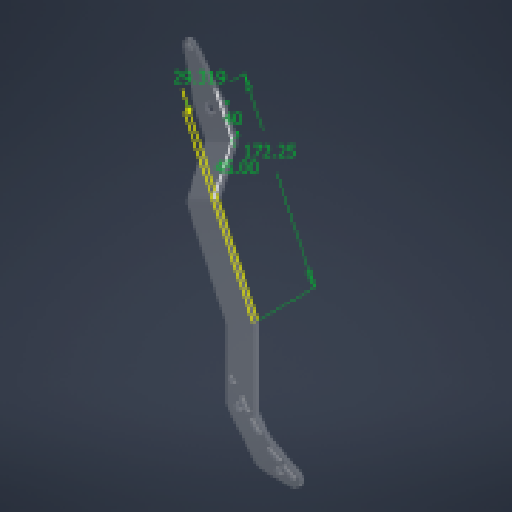
# Autodesk Inventor part: INTAKE_DROPPER_PLATE_SIDE
Saved by Autodesk Inventor 2026.2 (Build 302298010, 298A)
## iProperties
Created: 2026-04-03
Part Number: INTAKE_DROPPER_PLATE_SIDE
Material: Polycarbonate, Clear
Document SubType Name: Sheet Metal
Designer: 4aida
Density: 1.2 g/cm^3
Sheet Metal Rule: Default_mm
Appearance: Polycarbonate - Clear
Author: 4aida
Autodesk Inventor part; units mm, degrees
ref_plane "YZ Plane" through (0, 0, 0) normal (1, 0, 0) x (0, 1, 0)
ref_plane "XZ Plane" through (0, 0, 0) normal (0, 1, 0) x (-1, 0, 0)
ref_plane "XY Plane" through (0, 0, 0) normal (0, 0, 1) x (1, 0, 0)
sketch "Sketch6" plane through (5.547, -11.9185, -29.5428) normal (-0.0007043, -0.0003281, 0.9999997) x (0.9064037, 0.4224119, 0.0007769)
  circle A0 centre (0, 50) radius 3
  circle A1 centre (0, 50) radius 6
  line L0 (5.8818, 51.185) -> (16.194, 0)
  line L1 (16.194, 0) -> (-16.194, 0)
  line L2 (-16.194, 0) -> (-5.8818, 51.185)
  arc A2 (15.875, 0.0087) -> (-15.875, 0.0087) centre (0, 0) ccw
  point P0 (0.0297, 13.1461)
  point P1 (-15.5623, 3.1353)
  point P2 (15.5623, 3.1353)
  dimension "d68" = 6
  dimension "d69" = 12
  dimension "d70" = 50
  measures "d68" diameter of A0
  measures "d69" diameter of A1
  measures "d70" distance of A2.centre A0.centre
sketch "Sketch1" plane through (0, 0, 0) normal (0, 0, 1) x (1, 0, 0)
  circle A0 centre (0, 0) radius 2.4384
  circle A1 centre (0, 0) radius 15.875
  line L0 (-14.395, -6.6933) -> (56.9691, -160.1742)
  line L1 (90.6025, -274.8968) -> (130.7528, -274.8968)
  line L2 (86.9691, -148.9425) -> (14.3876, 6.7091)
  line L3 (129.6597, -266.3023) -> (96.0194, -248.4154)
  line L4 (96.0194, -248.4154) -> (72.0423, -218.8061)
  line L5 (72.0423, -218.8061) -> (69.5749, -220.8042) construction
  line L6 (69.5749, -220.8042) -> (93.9585, -250.9155)
  line L7 (93.9585, -250.9155) -> (128.1691, -269.1056)
  line L8 (128.1691, -269.1056) -> (129.6597, -266.3023) construction
  line L9 (74.4494, -236.9141) -> (67.2074, -238.0611)
  line L10 (67.2074, -238.0611) -> (62.593, -232.3628)
  line L11 (62.593, -232.3628) -> (65.2206, -225.5175)
  line L12 (65.2206, -225.5175) -> (72.4627, -224.3704)
  line L13 (72.4627, -224.3704) -> (77.0771, -230.0687) construction
  line L14 (77.0771, -230.0687) -> (74.4494, -236.9141)
  line L15 (112.0091, -274.8968) -> (105.535, -271.4545)
  line L16 (105.535, -271.4545) -> (105.2791, -264.1266)
  line L17 (105.2791, -264.1266) -> (111.4973, -260.2411)
  line L18 (111.4973, -260.2411) -> (117.9714, -263.6834) construction
  line L19 (117.9714, -263.6834) -> (118.2273, -271.0113)
  line L20 (118.2273, -271.0113) -> (112.0091, -274.8968)
  line L21 (128.1691, -269.1056) -> (106.6818, -269.1056) construction
  line L22 (5.0853, -149.4208) -> (51.9691, -149.4208) construction
  line L23 (51.9691, -149.4208) -> (51.9691, -259.6568) construction
  line L24 (51.9691, -259.6568) -> (5.0853, -259.6568) construction
  line L25 (5.0853, -259.6568) -> (5.0853, -149.4208) construction
  line L26 (-7.7017, -21.0883) -> (-3.3832, -19.0803)
  line L27 (-1.2744, -19.8505) -> (-1.2744, -19.8505)
  line L28 (-2.0446, -21.9593) -> (-6.3631, -23.9673)
  arc A2 (-1.2744, -19.8505) -> (-3.3832, -19.0803) centre (-2.7139, -20.5198) ccw
  arc A3 (-2.0446, -21.9593) -> (-1.2744, -19.8505) centre (-2.7139, -20.5198) ccw
  line L29 (130.7528, -274.8968) -> (136.4218, -264.2349)
  line L30 (136.4218, -264.2349) -> (99.265, -244.4782)
  line L31 (99.265, -244.4782) -> (86.9691, -229.2942)
  line L32 (86.9691, -229.2942) -> (86.9691, -148.9425)
  line L33 (56.9691, -160.1742) -> (56.9691, -233.363)
  line L34 (56.9691, -233.363) -> (90.6025, -274.8968)
  circle A4 centre (69.835, -231.2158) radius 3.175
  circle A5 centre (111.7532, -267.569) radius 3.175
  line L35 (74.0404, -221.2736) -> (71.573, -223.2717) construction
  line L36 (80.3336, -229.045) -> (77.8662, -231.0431) construction
  line L37 (125.3658, -267.6151) -> (126.8564, -264.8117) construction
  line L38 (118.0269, -260.117) -> (116.5363, -262.9203) construction
  line L39 (102.6084, -251.9188) -> (101.1178, -254.7222) construction
  line L40 (111.4379, -256.6136) -> (109.9473, -259.4169) construction
  line L41 (91.3231, -242.616) -> (88.8557, -244.6141) construction
  line L42 (85.0299, -234.8445) -> (82.5625, -236.8426) construction
  arc A6 (125.3658, -267.6151) -> (126.8564, -264.8117) centre (126.1111, -266.2134) ccw
  arc A7 (118.0269, -260.117) -> (116.5363, -262.9203) centre (117.2816, -261.5187) ccw
  arc A8 (109.9473, -259.4169) -> (111.4379, -256.6136) centre (110.6926, -258.0152) ccw
  arc A9 (102.6084, -251.9188) -> (101.1178, -254.7222) centre (101.8631, -253.3205) ccw
  arc A10 (88.8557, -244.6141) -> (91.3231, -242.616) centre (90.0894, -243.615) ccw
  arc A11 (85.0299, -234.8445) -> (82.5625, -236.8426) centre (83.7962, -235.8435) ccw
  arc A12 (77.8662, -231.0431) -> (80.3336, -229.045) centre (79.0999, -230.0441) ccw
  arc A13 (74.0404, -221.2736) -> (71.573, -223.2717) centre (72.8067, -222.2726) ccw
  circle A14 centre (63.3191, -209.7457) radius 3.175
  line L43 (0, 0) -> (5.5633, -11.9306) construction
  point P0 (-22.2711, -102.6289)
  point P1 (52.3674, -261.3253)
  point P2 (-1.2744, -19.8505)
  point P3 (111.4973, -260.2411)
  dimension "d0" = 38.1
  dimension "d1" = 38.1
  dimension "d2" = 157
  dimension "d3" = 3.175
  dimension "d4" = 3.175
  dimension "d5" = 76.2
  dimension "d6" = 12.7
  dimension "d7" = 12.7
  dimension "d8" = 8.255
  dimension "d10" = 4.8768
  dimension "d11" = 31.75
  dimension "d14" = 28
  dimension "d15" = 76.2
  dimension "d16" = 125.476
  dimension "d19" = 65
  dimension "d21" = 6.35
  dimension "d22" = 3.175
  dimension "d23" = 1.5875
  dimension "d24" = 5
  dimension "d25" = 5
  dimension "d26" = 5
  dimension "d27" = 5
  dimension "d28" = 30
  dimension "d29" = 5
  dimension "d32" = 6.35
  dimension "d33" = 6.35
  dimension "d34" = 3.175
  dimension "d35" = 10
  dimension "d36" = 10
  dimension "d37" = 7.4625
  dimension "d38" = 7.4625
  dimension "d39" = 7.4625
  dimension "d40" = 10
  dimension "d41" = 7.4625
  dimension "d42" = 10
  dimension "d43" = 6.35
  dimension "d44" = 6.35
  dimension "d45" = 15.875
  dimension "d64" = 13.164
  dimension "d65" = 257.175
  dimension "d66" = 137.4902
  dimension "d67" = 122.6058
  measures "d0" distance of L3.end L4.end
  measures "d1" distance of L8.end L3.end
  measures "d2" angle of L3 L4
  measures "d3" distance of L4.end L6.start
  measures "d4" distance of L8.start L8.end
  measures "d5" distance of point (52.367, -261.325) L8.start
  measures "d6" distance between parallel lines of L10 L13
  measures "d7" distance between parallel lines of L18 L15
  measures "d8" distance from line of L5 point (69.835, -231.216)
  measures "d10" diameter of A0
  measures "d11" diameter of A1
  measures "d14" angle of L7 L21
  measures "d15" distance from line of L8.start L23
  measures "d16" distance between parallel lines of L1 L22
  measures "d19" angle of L2 L1
  measures "d21" distance between parallel lines of L27 L0
  measures "d22" distance between parallel lines of L28 L26
  measures "d23" radius of A2
  measures "d24" distance between parallel lines of L30 L3
  measures "d25" distance between parallel lines of L29 L8
  measures "d26" distance between parallel lines of L31 L4
  measures "d27" distance between parallel lines of L33 L23
  measures "d28" distance between parallel lines of L33 L32
  measures "d29" distance between parallel lines of L10 L34
  measures "d32" diameter of A4
  measures "d33" diameter of A5
  measures "d34" distance between parallel lines of L5 L35
  measures "d35" distance between parallel lines of L35 L36
  measures "d36" distance between parallel lines of L41 L42
  measures "d37" distance between parallel lines of L42 L36
  measures "d38" distance from line of L3.end L39
  measures "d39" distance from line of L3.end L41
  measures "d40" distance between parallel lines of L40 L39
  measures "d41" distance between parallel lines of L38 L40
  measures "d42" distance between parallel lines of L37 L38
  measures "d43" diameter of A14
  measures "d44" distance from line of A14.centre L33
  measures "d45" distance from line of L12 A14.centre
  measures "d64" distance of L43.start L43.end
  measures "d65" vertical distance of L43.end L8.start
  measures "d66" distance from line of L22 L43.end
  measures "d67" horizontal distance of L43.end L8.start
extrude "Plate1" add sketch "Sketch1" along normal blind 4.7625 contours A1 | L15 L16 L17 L7 L19 L20 | A1 L2 L32 L31 L30 L29 L1 L34 L33 L0 L28 A3 A2 L26 | L26 A2 A3 L28 L0 | L7 A8 L3 A7 | L7 L6 A10 L4 L3 A9 | L6 A12 L4 A11 | L14 L9 L10 L11 L12 L6
fillet "Corner Round1" radius 6 2 edges at (136.4218, -264.2349, 2.3813) (130.7528, -274.8968, 2.3813)
fillet "Corner Round1" radius 10 6 edges at (90.6025, -274.8968, 2.3813) (56.9691, -233.363, 2.3813) (99.265, -244.4782, 2.3813) (86.9691, -229.2942, 2.3813) (86.9691, -148.9425, 2.3813) (56.9691, -160.1742, 2.3813)
sketch "Sketch2" plane through (14.3876, 6.7091, 4.7625) normal (0.9063078, 0.4226183, 0) x (0, 0, -1)
  line L0 (0, 0) -> (0, -169.5255) projected
  line L1 (0, -71.3575) -> (34.082, -37.2755)
  line L2 (34.082, -37.2755) -> (34.082, 2.7245)
  line L3 (4.7625, -169.5255) -> (4.7625, 0) projected
  line L4 (4.7625, 15.875) -> (4.7625, 0) projected
  point P0 (4.7625, 0.0174)
  dimension "d46" = 29.3195
  dimension "d47" = 172.25
  dimension "d49" = 40
  dimension "d50" = 45
  constraints: 4 end point, 1 parallel, 1 point on line
  measures "d46" distance between parallel lines of L2 L3
  measures "d47" vertical distance of L3.start L2.end
  measures "d49" distance of L1.end L2.end
  measures "d50" angle of L2 L1
sketch "Sketch3" plane through (0, 0, 4.7625) normal (0, 0, 1) x (1, 0, 0)
  line L0 (14.3876, 6.7091) -> (86.0322, -146.9333) projected
  line L1 (44.5446, -57.9628) -> (15.6983, -71.4141)
  line L2 (56.0369, -158.1692) -> (-14.395, -6.6933) projected
  point P0 (0, 0)
  constraints: 3 point on line, 2 end point, 1 perpendicular
fold "Fold1" angle 45 bend radius 4.7625 thickness 4.7625 k factor 0.44 line from (44.5446, -57.9628, 4.7625) to (15.6983, -71.4141, 4.7625) line at bend end moving side (-0.4226183, 0.9063078, 0) folds toward (0, 0, -1)
sketch "Sketch4" plane through (15.1282, -70.1915, 1.9727) normal (-0.2988362, 0.6408564, 0.7071068) x (0.9066356, 0.4219139, 0.0007769)
  line L0 (31.7787, 45.3076) -> (0, 45.3076)
  line L1 (0, 0) -> (0, 71.375) projected
  point P0 (15.8975, 50.9159)
  constraints: 2 end point, 1 horizontal, 1 point on line
fold "Fold2" angle 45 bend radius 4.7625 thickness 4.7625 k factor 0.44 line from (30.4454, -27.727, -30.0399) to (1.6338, -41.1348, -30.0646) line at bend centre moving side (-0.2978403, 0.6413203, -0.7071064) folds toward (-0.2988362, 0.6408564, 0.7071068)
sheet face with bend "Face2" sketch "Sketch6" thickness 4.7625 toward (0.0007043, 0.0003281, -0.9999997) bend radius 4.7625 contours A1 | A1 L0 A2 L2
bend "Bend1"
equation "\"BendRadius\" = Thickness"
equation "\"BendReliefWidth\" = Thickness"
equation "\"BendReliefDepth\" = 0.5 * Thickness"
equation "\"CornerReliefSize\" = 4 * Thickness"
equation "\"MinimumRemnant\" = 2 * Thickness"
equation "\"TransitionRadius\" = BendRadius"
equation "\"JacobiRadiusSize\" = BendRadius"
equation "\"GapSize\" = Thickness"
equation "\"Thickness\" = 4.7625"
body "Solid1"
